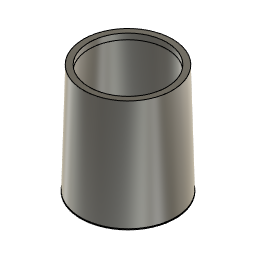
24wp_16.4-14.4_diameter_test_cone_open v2 (Autodesk Fusion 360 design; units mm, degrees)
Autodesk Fusion 360 part; units mm, degrees
note: some values were not read from the file. Set by a fixed rule: which face or edge a step refers to.
sketch "Sketch1" plane through (0, 0, 0) normal (0, 0, 1) x (1, 0, 0)
  circle A0 centre (0, 0) radius 8.2
  dimension "d1" = 16.4
  constraint coincident A0.centre origin
  measures "d1" diameter of A0
extrude "Extrude1" add sketch "Sketch1" along normal blind 19
chamfer "Chamfer1" distance 0.5 angle 88.48 1 edges at (-7.6451, -2.9652, 19) measured on face at (1.6133, 1.7387, 19)
shell "Shell1" thickness 1 removed faces 1 at (1.6133, 1.7387, 0)
extrude "Extrude2" cut 1 faces at (-3.862, -0.2442, 18) along direction (0, 0, 1) blind 1
